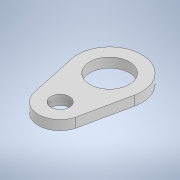
# Autodesk Inventor part: palanca2
Saved by Autodesk Inventor 2021 (Build 250183000, 183)
## iProperties
Created: 2026-06-16
Part Number: palanca2
Material: Generic
Document SubType Name: Sheet Metal
Designer: nelso
Density: 1 g/cm^3
Sheet Metal Rule: Default_mm
Appearance: Default
Author: nelso
Autodesk Inventor part; units mm, degrees
ref_plane "YZ Plane" through (0, 0, 0) normal (1, 0, 0) x (0, 1, 0)
ref_plane "XZ Plane" through (0, 0, 0) normal (0, 1, 0) x (-1, 0, 0)
ref_plane "XY Plane" through (0, 0, 0) normal (0, 0, 1) x (1, 0, 0)
sketch "Sketch1" plane through (0, 0, 0) normal (0, 1, 0) x (-1, 0, 0)
  circle A0 centre (1.7771, 6.2477) radius 3
  circle A1 centre (1.8209, -9.7522) radius 6.35
  circle A2 centre (1.7771, 6.2477) radius 7
  circle A3 centre (1.8209, -9.7522) radius 10.35
  line L0 (8.6179, 7.732) -> (11.9355, -7.5575)
  line L1 (-5, 8) -> (-8.3047, -7.6084)
  point P0 (0, 0)
  dimension "d3" = 6
  dimension "d5" = 12.7
  dimension "d6" = 14
  dimension "d7" = 20.7
  dimension "d8" = 16
  measures "d3" diameter of A0
  measures "d5" diameter of A1
  measures "d6" diameter of A2
  measures "d7" diameter of A3
  measures "d8" distance of A1.centre A0.centre
extrude "Plate1" add sketch "Sketch1" along normal mid plane 3.1 contours A2 A3 L1 | A2 L0 A3 | A3 A2 | A2 A3 | A3 L1 A2
equation "\"d9\" = Thickness"
equation "\"BendRadius\" = Thickness"
equation "\"BendReliefWidth\" = Thickness"
equation "\"BendReliefDepth\" = 0.5 * Thickness"
equation "\"CornerReliefSize\" = 4 * Thickness"
equation "\"MinimumRemnant\" = 2 * Thickness"
equation "\"TransitionRadius\" = BendRadius"
equation "\"JacobiRadiusSize\" = BendRadius"
equation "\"GapSize\" = Thickness"
equation "\"Thickness\" = 3.1"
body "Solid1"
